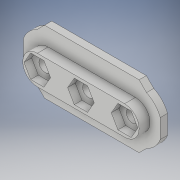
# Autodesk Inventor part: NerfBottomInsert
Saved by Autodesk Inventor 2018.3 (Build 223284000, 284)
## iProperties
Created: 2019-08-17
Part Number: NerfBottomInsert
Material: Generic
Document SubType Name: Modeling
Designer: Srinity
Density: 1 g/cm^3
Appearance: Default
Author: Srinity
Autodesk Inventor part; units mm, degrees
ref_plane "YZ Plane" through (0, 0, 0) normal (1, 0, 0) x (0, 1, 0)
ref_plane "XZ Plane" through (0, 0, 0) normal (0, 1, 0) x (-1, 0, 0)
ref_plane "XY Plane" through (0, 0, 0) normal (0, 0, 1) x (1, 0, 0)
sketch "Sketch1" plane through (0, 0, 0) normal (0, 0, 1) x (1, 0, 0)
  line L0 (-19.575, 13.075) -> (19.575, 13.075)
  line L1 (19.575, 13.075) -> (19.575, -13.075)
  line L2 (19.575, -13.075) -> (-19.575, -13.075)
  line L3 (-19.575, -13.075) -> (-19.575, 13.075)
  circle A0 centre (-18.075, 0) radius 5.8 construction
  circle A1 centre (18.075, 0) radius 5.8 construction
  line L4 (-23.875, 6.8771) -> (-23.875, -8.4899) construction
  line L5 (23.875, 6.9073) -> (23.875, -5.3677) construction
  arc A2 (-28.35, -3.9274) -> (-28.35, 3.9274) centre (-18.075, 0) ccw
  arc A3 (28.35, 3.9274) -> (28.35, -3.9274) centre (18.075, 0) ccw
  line L6 (-28.35, 3.9274) -> (-28.35, -3.9274)
  line L7 (28.35, -3.9274) -> (28.35, 3.9274)
  arc A4 (-28.35, 3.9274) -> (-28.35, -3.9274) centre (-18.075, 0) ccw
  arc A5 (28.35, -3.9274) -> (28.35, 3.9274) centre (18.075, 0) ccw
  line L8 (-19.575, 13.075) -> (-22.6436, 10.0064)
  line L9 (-19.575, -13.075) -> (-22.6436, -10.0064)
  line L10 (19.575, -13.075) -> (22.6436, -10.0064)
  line L11 (19.575, 13.075) -> (22.6436, 10.0064)
  point P0 (0, 0)
  dimension "d0" = 39.15
  dimension "d1" = 19.575
  dimension "d2" = 26.15
  dimension "d3" = 13.075
  dimension "d4" = 11.6
  dimension "d5" = 47.75
  dimension "d6" = 23.875
  dimension "d7" = 22
  dimension "d8" = 56.7
  dimension "d9" = 28.35
  dimension "d10" = 135
  constraints: 24 end point, 12 point on circle, 6 centre point, 4 perpendicular, 3 parallel, 3 vertical, 2 coincident, 2 equal radius, 2 horizontal alignment, 2 tangent, 1 horizontal
  measures "d0" distance of L0.start L0.end
  measures "d1" distance from line of point (0, 0) L3
  measures "d2" distance between parallel lines of L2 L0
  measures "d3" distance from line of point (0, 0) L0
  measures "d4" diameter of A0
  measures "d5" distance between parallel lines of L5 L4
  measures "d6" distance from line of point (0, 0) L4
  measures "d7" diameter of A2
  measures "d8" distance between parallel lines of L7 L6
  measures "d9" distance from line of point (0, 0) L6
  measures "d10" angle of L11 L0
extrude "Extrusion1" add sketch "Sketch1" along normal blind 3 contours L0 L1 A3 L2 L3 A2 | L3 A2 L8 | L11 A3 L1 | A2 L3 | L3 A2 L6 | A3 L7 L1 | L1 A3 | L3 L9 A2 | A3 L10 L1
sketch "Sketch2" plane through (0, 0, 3) normal (0, 0, 1) x (1, 0, 0)
  circle A0 centre (-18.075, 0) radius 6
  circle A1 centre (18.075, 0) radius 6
  arc A2 (28.35, 3.9274) -> (22.6436, 10.0064) centre (18.075, 0) ccw projected
  arc A3 (-22.6436, 10.0064) -> (-28.35, 3.9274) centre (-18.075, 0) ccw projected
  line L0 (-18.075, 6) -> (18.075, 6)
  line L1 (18.075, 6) -> (18.075, -6)
  line L2 (18.075, -6) -> (-18.075, -6)
  line L3 (-18.075, -6) -> (-18.075, 6)
  point P0 (0, 0)
  dimension "d13" = 12
  constraints: 8 end point, 2 centre point, 2 concentric, 2 midpoint, 2 parallel, 2 tangent, 1 equal radius, 1 horizontal, 1 perpendicular
  measures "d13" diameter of A0
extrude "Extrusion2" add sketch "Sketch2" along normal blind 4.5
sketch "Sketch3" plane through (0, 0, 7.5) normal (0, 0, 1) x (1, 0, 0)
  circle A0 centre (-18.075, 0) radius 2.4892
  circle A1 centre (18.075, 0) radius 2.4892
  circle A2 centre (0, 0) radius 2.4892
  arc A3 (-18.075, 6) -> (-18.075, -6) centre (-18.075, 0) ccw projected
  arc A4 (18.075, -6) -> (18.075, 6) centre (18.075, 0) ccw projected
  line L0 (-20.8246, 4.7625) -> (-15.3254, 4.7625)
  line L1 (-15.3254, 4.7625) -> (-12.5757, 0)
  line L2 (-12.5757, 0) -> (-15.3254, -4.7625)
  line L3 (-15.3254, -4.7625) -> (-20.8246, -4.7625)
  line L4 (-20.8246, -4.7625) -> (-23.5743, 0)
  line L5 (-23.5743, 0) -> (-20.8246, 4.7625)
  line L6 (-2.7496, 4.7625) -> (2.7496, 4.7625)
  line L7 (2.7496, 4.7625) -> (5.4993, 0)
  line L8 (5.4993, 0) -> (2.7496, -4.7625)
  line L9 (2.7496, -4.7625) -> (-2.7496, -4.7625)
  line L10 (-2.7496, -4.7625) -> (-5.4993, 0)
  line L11 (-5.4993, 0) -> (-2.7496, 4.7625)
  line L12 (15.3254, 4.7625) -> (20.8246, 4.7625)
  line L13 (20.8246, 4.7625) -> (23.5743, 0)
  line L14 (23.5743, 0) -> (20.8246, -4.7625)
  line L15 (20.8246, -4.7625) -> (15.3254, -4.7625)
  line L16 (15.3254, -4.7625) -> (12.5757, 0)
  line L17 (12.5757, 0) -> (15.3254, 4.7625)
  dimension "d16" = 4.9784
  dimension "d17" = 9.525
  constraints: 36 end point, 4 coincident, 4 collinear, 3 centre point, 2 concentric, 2 equal radius, 2 horizontal alignment, 39 other
  measures "d16" diameter of A0
  measures "d17" distance between parallel lines of L3 L0
extrude "Extrusion3" cut sketch "Sketch3" against normal through all contours A0 | A1 | A2
sketch "Sketch4" plane through (0, 0, 7.5) normal (0, 0, 1) x (1, 0, 0)
  circle A0 centre (-18.075, 0) radius 2.4892 projected
  line L0 (-15.3254, 4.7625) -> (-12.5757, 0)
  line L1 (-12.5757, 0) -> (-15.3254, -4.7625)
  line L2 (-15.3254, -4.7625) -> (-20.8246, -4.7625)
  line L3 (-20.8246, -4.7625) -> (-23.5743, 0)
  line L4 (-23.5743, 0) -> (-20.8246, 4.7625)
  line L5 (-20.8246, 4.7625) -> (-15.3254, 4.7625)
  circle A1 centre (0, 0) radius 2.4892 projected
  line L6 (2.7496, 4.7625) -> (5.4993, 0)
  line L7 (5.4993, 0) -> (2.7496, -4.7625)
  line L8 (2.7496, -4.7625) -> (-2.7496, -4.7625)
  line L9 (-2.7496, -4.7625) -> (-5.4993, 0)
  line L10 (-5.4993, 0) -> (-2.7496, 4.7625)
  line L11 (-2.7496, 4.7625) -> (2.7496, 4.7625)
  circle A2 centre (18.075, 0) radius 2.4892 projected
  line L12 (15.3254, 4.7625) -> (20.8246, 4.7625)
  line L13 (20.8246, 4.7625) -> (23.5743, 0)
  line L14 (23.5743, 0) -> (20.8246, -4.7625)
  line L15 (20.8246, -4.7625) -> (15.3254, -4.7625)
  line L16 (15.3254, -4.7625) -> (12.5757, 0)
  line L17 (12.5757, 0) -> (15.3254, 4.7625)
  dimension "d20" = 9.525
  constraints: 36 end point, 3 coincident, 3 collinear, 39 other
  measures "d20" distance between parallel lines of L2 L5
extrude "Extrusion4" cut sketch "Sketch4" against normal blind 3.175 contours A0 | L0 L1 L2 L3 L4 L5 | A1 | L6 L7 L8 L9 L10 L11 | A2 | L12 L13 L14 L15 L16 L17
equation "\"d1\" = 0.5 * d0"
equation "\"d3\" = 0.5 * d2"
equation "\"d6\" = 0.5 * d5"
equation "\"d9\" = 0.5 * d8"
body "Solid1"
